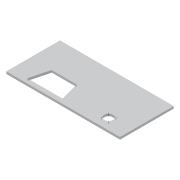
# Autodesk Inventor part: Lid_TopPanel2
Saved by Autodesk Inventor 2016 (Build 200138000, 138)
## iProperties
Created: 2014-10-15
Part Number: Lid_TopPanel2
Material: Polycarbonat, klar
Document SubType Name: Modeling
Designer: Gero Hofmann
Density: 1.2 g/cm^3
Appearance: Polycarbonat - klar
Author: Gero Hofmann
Autodesk Inventor part; units mm, degrees
ref_plane "YZ Plane" through (0, 0, 0) normal (1, 0, 0) x (0, 1, 0)
ref_plane "XZ Plane" through (0, 0, 0) normal (0, 1, 0) x (-1, 0, 0)
ref_plane "XY Plane" through (0, 0, 0) normal (0, 0, 1) x (1, 0, 0)
sketch "Skizze1" plane through (0, 0, 0) normal (0, 0, 1) x (1, 0, 0)
  line L0 (-250, 120) -> (250, 120)
  line L1 (250, 120) -> (250, -120)
  line L2 (250, -120) -> (-250, -120)
  line L3 (-250, -120) -> (-250, 120)
  line L4 (-250, 120) -> (250, -120) construction
  line L5 (250, 120) -> (-250, -120) construction
  point P0 (0, 0)
  dimension "d0" = 500
  dimension "d1" = 240
  constraints: 12 end point, 2 midpoint, 2 parallel, 1 horizontal, 1 perpendicular
  measures "d0" distance of L1.end L2.end
  measures "d1" distance of L0.end L1.end
extrude "Extrusion1" add sketch "Skizze1" along normal blind 10
sketch "Skizze2" plane through (0, 0, 10) normal (0, 0, 1) x (1, 0, 0)
  line L0 (-250, 120) -> (-250, -120) projected
  line L1 (-250, -120) -> (250, -120) projected
  line L2 (250, -120) -> (250, 120) projected
  line L3 (-177.5, -100) -> (-155, -15)
  line L4 (-155, -15) -> (-45, -15)
  line L5 (-45, -15) -> (-22.5, -100)
  line L6 (-177.5, -100) -> (-22.5, -100)
  line L7 (143.755, -89) -> (156.245, -89)
  line L8 (169, -76.245) -> (169, -63.755)
  line L9 (156.245, -51) -> (143.755, -51)
  line L10 (131, -63.755) -> (131, -76.245)
  line L11 (143.755, -89) -> (156.245, -51) construction
  line L12 (169, -76.245) -> (131, -63.755) construction
  arc A0 (156.245, -89) -> (169, -76.245) centre (150, -70) ccw
  arc A1 (131, -76.245) -> (143.755, -89) centre (150, -70) ccw
  arc A2 (169, -63.755) -> (156.245, -51) centre (150, -70) ccw
  arc A3 (143.755, -51) -> (131, -63.755) centre (150, -70) ccw
  point P0 (0, 0)
  point P1 (-100, -15)
  point P2 (-100, -100)
  point P3 (-33.75, -57.5)
  dimension "d25" = 155
  dimension "d26" = 110
  dimension "d27" = 150
  dimension "d28" = 20
  dimension "d29" = 85
  dimension "d33" = 100
  dimension "d34" = 50
  dimension "d47" = 38
  dimension "d48" = 20
  constraints: 20 end point, 8 point on circle, 5 midpoint, 4 centre point, 3 concentric, 3 parallel, 3 perpendicular, 1 horizontal, 1 vertical alignment
  measures "d25" distance of L3.start L5.end
  measures "d26" distance of L3.end L4.end
  measures "d27" distance from line of L0 point (-100, -100)
  measures "d28" distance between parallel lines of L1 L6
  measures "d29" distance between parallel lines of L6 L4
  measures "d33" distance from line of L2 A0.centre
  measures "d34" distance from line of L1 A0.centre
  measures "d47" distance between parallel lines of L7 L9
  measures "d48" radius of A2
extrude "Extrusion2" cut sketch "Skizze2" against normal blind 10
sketch "Skizze3" plane through (0, 0, 10) normal (0, 0, 1) x (1, 0, 0)
  circle A0 centre (150, -70) radius 20 projected
  line L0 (134, -86) -> (166, -86)
  line L1 (166, -86) -> (166, -54)
  line L2 (166, -54) -> (134, -54)
  line L3 (134, -54) -> (134, -86)
  line L4 (134, -86) -> (166, -54) construction
  line L5 (166, -86) -> (134, -54) construction
  point P0 (0, 0)
  dimension "d35" = 32
  dimension "d36" = 32
  constraints: 12 end point, 2 midpoint, 2 parallel, 1 horizontal, 1 perpendicular
  measures "d35" distance of L2.end L1.end
  measures "d36" distance of L1.end L0.end
hole "Bohrung3" at (166, -54, 10) at (134, -54, 10) at (134, -86, 10) at (166, -86, 10) direction (0, 0, -1) diameter 2.459 end through all thread size "M3x0.5" class "6H" standard "ISO Metric profile"
